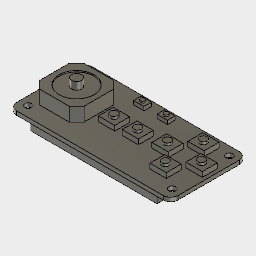
3464 Joy Bonnet (Autodesk Fusion 360 design; units mm, degrees)
Autodesk Fusion 360 part; units mm, degrees
sketch "Adafruit Joy Bonnet" plane through (0, 0, 0) normal (0, 0, 1) x (1, 0, 0)
  line L0 (33.9045, 27.9414) -> (38.1045, 27.9414)
  circle A0 centre (36.0045, 14.986) radius 1.5033
  circle A1 centre (53.34, 24.13) radius 1.5033
  line L1 (56.64, 21.13) -> (50.04, 21.13)
  line L2 (56.64, 25.33) -> (56.64, 22.93)
  line L3 (50.04, 11.89) -> (56.64, 11.89)
  line L4 (50.04, 22.93) -> (50.04, 25.33)
  line L5 (32.7045, 13.786) -> (32.7045, 16.186)
  line L6 (23.1795, 17.986) -> (29.7795, 17.986)
  line L7 (5.43, 5.986) -> (2.43, 8.986)
  circle A2 centre (36.0045, 14.986) radius 1
  line L8 (39.3045, 16.186) -> (39.3045, 13.786)
  line L9 (43.182, 15.31) -> (43.182, 17.71)
  line L10 (43.182, 19.51) -> (49.782, 19.51)
  line L11 (20.43, 20.986) -> (20.43, 8.986)
  line L12 (49.782, 13.51) -> (43.182, 13.51)
  line L13 (2.43, 8.986) -> (2.43, 20.986)
  line L14 (50.04, 27.13) -> (56.64, 27.13)
  circle A3 centre (46.482, 16.51) radius 1
  circle A4 centre (53.34, 24.13) radius 1
  line L15 (32.7045, 17.986) -> (39.3045, 17.986)
  circle A5 centre (11.43, 14.986) radius 7
  line L16 (39.3045, 11.986) -> (32.7045, 11.986)
  line L17 (17.43, 5.986) -> (5.43, 5.986)
  line L18 (20.43, 8.986) -> (17.43, 5.986)
  circle A6 centre (26.4795, 14.986) radius 1
  line L19 (29.7795, 16.186) -> (29.7795, 13.786)
  line L20 (2.43, 20.986) -> (5.43, 23.986)
  line L21 (17.43, 23.986) -> (20.43, 20.986)
  line L22 (5.43, 23.986) -> (17.43, 23.986)
  circle A7 centre (26.4795, 14.986) radius 1.5033
  line L23 (23.1795, 13.786) -> (23.1795, 16.186)
  line L24 (56.898, 15.31) -> (56.898, 17.71)
  circle A8 centre (60.198, 16.51) radius 1.5033
  circle A9 centre (60.198, 16.51) radius 1
  line L25 (29.7795, 11.986) -> (23.1795, 11.986)
  line L26 (63.498, 13.51) -> (56.898, 13.51)
  circle A10 centre (53.34, 8.89) radius 1
  line L27 (63.498, 17.71) -> (63.498, 15.31)
  line L28 (56.898, 19.51) -> (63.498, 19.51)
  line L29 (24.3795, 28.0049) -> (28.5795, 28.0049)
  line L30 (28.5795, 24.9541) -> (24.3795, 24.9541)
  line L31 (38.1045, 24.8906) -> (33.9045, 24.8906)
  line L32 (56.64, 5.89) -> (50.04, 5.89)
  line L33 (56.64, 10.09) -> (56.64, 7.69)
  line L34 (50.04, 7.69) -> (50.04, 10.09)
  circle A11 centre (53.34, 8.89) radius 1.5033
  circle A12 centre (46.482, 16.51) radius 1.5033
  line L35 (49.782, 17.71) -> (49.782, 15.31)
  arc A13 (61.9605, -0.6884) -> (64.9605, 2.3116) centre (61.9605, 2.3116) ccw
  circle A14 centre (3.4605, 3.472) radius 1.4
  arc A15 (2.9605, 29.972) -> (-0.0395, 26.972) centre (2.9605, 26.972) ccw
  line L36 (61.9605, 29.972) -> (2.9605, 29.972)
  line L37 (-0.0395, 26.972) -> (-0.0395, 2.3116)
  arc A16 (64.9605, 26.972) -> (61.9605, 29.972) centre (61.9605, 26.972) ccw
  line L38 (64.9605, 2.3116) -> (64.9605, 26.972)
  arc A17 (-0.0395, 2.3116) -> (2.9605, -0.6884) centre (2.9605, 2.3116) ccw
  line L39 (2.9605, -0.6884) -> (61.9605, -0.6884)
  circle A18 centre (61.4605, 26.472) radius 1.4
  circle A19 centre (61.4605, 3.472) radius 1.4
  circle A20 centre (3.4605, 26.472) radius 1.4
  line L40 (57.8485, -0.508) -> (57.8485, 3.556)
  line L41 (55.3085, -0.508) -> (57.8485, -0.508)
  line L42 (7.0485, 7.366) -> (7.0485, -0.508)
  line L43 (57.8485, 3.556) -> (57.8485, 7.366)
  line L44 (7.0485, -0.508) -> (55.3085, -0.508)
  line L45 (57.8485, 7.366) -> (7.0485, 7.366)
  line L46 (50.04, 27.13) -> (56.64, 27.13)
  line L47 (56.64, 27.13) -> (56.64, 21.13)
  line L48 (56.64, 21.13) -> (50.04, 21.13)
  line L49 (50.04, 21.13) -> (50.04, 27.13)
  line L50 (56.898, 19.51) -> (63.498, 19.51)
  line L51 (63.498, 19.51) -> (63.498, 13.51)
  line L52 (63.498, 13.51) -> (56.898, 13.51)
  line L53 (56.898, 13.51) -> (56.898, 19.51)
  line L54 (50.04, 11.89) -> (56.64, 11.89)
  line L55 (56.64, 11.89) -> (56.64, 5.89)
  line L56 (56.64, 5.89) -> (50.04, 5.89)
  line L57 (50.04, 5.89) -> (50.04, 11.89)
  line L58 (43.182, 19.51) -> (49.782, 19.51)
  line L59 (49.782, 19.51) -> (49.782, 13.51)
  line L60 (49.782, 13.51) -> (43.182, 13.51)
  line L61 (43.182, 13.51) -> (43.182, 19.51)
  line L62 (32.7045, 17.986) -> (39.3045, 17.986)
  line L63 (39.3045, 17.986) -> (39.3045, 11.986)
  line L64 (39.3045, 11.986) -> (32.7045, 11.986)
  line L65 (32.7045, 11.986) -> (32.7045, 17.986)
  line L66 (23.1795, 17.986) -> (29.7795, 17.986)
  line L67 (29.7795, 17.986) -> (29.7795, 11.986)
  line L68 (29.7795, 11.986) -> (23.1795, 11.986)
  line L69 (23.1795, 11.986) -> (23.1795, 17.986)
  line L70 (24.3795, 28.0049) -> (28.5795, 28.0049)
  line L71 (28.5795, 28.0049) -> (28.5795, 24.9541)
  line L72 (28.5795, 24.9541) -> (24.3795, 24.9541)
  line L73 (24.3795, 24.9541) -> (24.3795, 28.0049)
  line L74 (33.9045, 27.9414) -> (38.1045, 27.9414)
  line L75 (38.1045, 27.9414) -> (38.1045, 24.8906)
  line L76 (38.1045, 24.8906) -> (33.9045, 24.8906)
  line L77 (33.9045, 24.8906) -> (33.9045, 27.9414)
  circle A21 centre (26.4795, 26.4795) radius 0.875
  circle A22 centre (36.0045, 26.416) radius 0.875
  circle A23 centre (11.43, 14.986) radius 2
  line L78 (0, 0) -> (5.5, 0)
  line L79 (0, 0) -> (0, 3.9)
  dimension "d1" = 1.75
  dimension "d2" = 1.75
  dimension "d14" = 4
  measures "d1" diameter of A21
  measures "d2" diameter of A22
  measures "d14" diameter of A23
extrude "Extrude1" add sketch "Adafruit Joy Bonnet" along normal blind 1.6 contours L0 L31 L74 L75 L76 L77 | A0 | A1 | L1 L2 L4 L14 L46 L47 L48 L49 | L3 L33 L34 L45 L54 L55 L57 | L17 L18 L32 L40 L41 L42 L43 L44 L45 L55 L56 L57 | L32 L45 L55 L56 L57 | L7 L11 L13 L17 L18 L20 L21 L22 L42 L45 | L17 L18 L42 L45 | L5 L8 L15 L16 L62 L63 L64 L65 | L6 L19 L23 L25 L66 L67 L68 L69 | A2 | L9 L10 L12 L35 L58 L59 L60 L61 | A3 | A4 | A5 | A6 | A7 | L24 L26 L27 L28 L50 L51 L52 L53 | A8 | A9 | A10 | L29 L30 L70 L71 L72 L73 | A11 | A12 | A13 A15 L36 L37 A16 L38 A17 L39 | A21 | A22 | A23
extrude "Extrude2" add sketch "Adafruit Joy Bonnet" along normal blind 2 from surface at 1.6 contours A0 | A1 | L1 L2 L4 L14 L46 L47 L48 L49 | L3 L33 L34 L45 L54 L55 L57 | L32 L45 L55 L56 L57 | L5 L8 L15 L16 L62 L63 L64 L65 | L6 L19 L23 L25 L66 L67 L68 L69 | A2 | L9 L10 L12 L35 L58 L59 L60 L61 | A3 | A4 | A6 | A7 | L24 L26 L27 L28 L50 L51 L52 L53 | A8 | A9 | A10 | A11 | A12
extrude "Extrude3" add sketch "Adafruit Joy Bonnet" along normal blind 1 from surface at 3.6 contours A0 | A1 | A2 | A3 | A4 | A6 | A7 | A8 | A9 | A10 | A11 | A12
extrude "Extrude4" add sketch "Adafruit Joy Bonnet" along normal blind 5.5 from surface at 1.6 contours L7 L11 L13 L17 L18 L20 L21 L22 L42 L45 | L17 L18 L42 L45 | A5 | A23
extrude "Extrude5" cut sketch "Adafruit Joy Bonnet" against normal blind 0.5 from surface at 7.1 contours A5 | A23
extrude "Extrude6" add sketch "Adafruit Joy Bonnet" along normal blind 3 from surface at 6.6 contours A23
extrude "Extrude7" add sketch "Adafruit Joy Bonnet" along normal blind 1.5 from surface at 1.6 contours L0 L31 L74 L75 L76 L77 | L29 L30 L70 L71 L72 L73 | A21 | A22
extrude "Extrude8" add sketch "Adafruit Joy Bonnet" along normal blind 0.6 from surface at 3.1 contours A21 | A22
extrude "Extrude9" add sketch "Adafruit Joy Bonnet" against normal blind 4.2 contours L17 L18 L32 L40 L41 L42 L43 L44 L45 L55 L56 L57 | L32 L45 L55 L56 L57 | L17 L18 L42 L45
move_face "OffsetFaces3" offset -1.437 2 faces at (40.9152, -0.508, -1.4) (23.9818, 7.366, -2.8)
move_body "Move1" bodies 1 to x (1, 0, 0) y (0, 1, 0) z (0, 0, 1) at (0.04, 0.688, 0)
equation "d31 = ( -2.874 / 2 ) * 1 mm"
